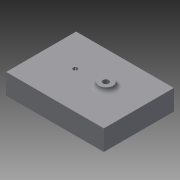
# Autodesk Inventor part: GehäuseFront
Saved by Autodesk Inventor 2014 (Build 180170000, 170)
## iProperties
Created: 2013-05-31
Part Number: GehäuseFront
Material: Generisch
Document SubType Name: Modeling
Designer: hanse
Density: 1 g/cm^3
Appearance: Vorgabe
Author: hanse
Autodesk Inventor part; units mm, degrees
ref_plane "YZ Plane" through (0, 0, 0) normal (1, 0, 0) x (0, 1, 0)
ref_plane "XZ Plane" through (0, 0, 0) normal (0, 1, 0) x (-1, 0, 0)
ref_plane "XY Plane" through (0, 0, 0) normal (0, 0, 1) x (1, 0, 0)
sketch "Skizze1" plane through (0, 0, 0) normal (0, 0, 1) x (1, 0, 0)
  line L0 (0, 0) -> (47.7997, 0)
  line L1 (47.7997, 0) -> (47.7997, 34.2455)
  line L2 (47.7997, 34.2455) -> (0, 34.2455)
  line L3 (0, 34.2455) -> (0, 0)
  circle A0 centre (15.5546, 18.2455) radius 1.05
  circle A1 centre (30.5546, 18.2455) radius 1.45
  line L4 (0, 18.2455) -> (47.7997, 18.2455)
  dimension "d0" = 2.1
  dimension "d1" = 2.9
  dimension "d2" = 15
  dimension "d16" = 16
  constraints: 10 end point, 4 point on line, 2 centre point, 2 parallel, 2 perpendicular, 1 horizontal
  measures "d0" diameter of A0
  measures "d1" diameter of A1
  measures "d2" distance of A1.centre A0.centre
  measures "d16" distance between parallel lines of L2 L4
extrude "Extrusion1" add sketch "Skizze1" along normal blind 2 contours L3 L4 A0 A1 L1 L0 | L3 L2 L1 L4 A1 A0
sketch "Skizze2" plane through (0, 0, 0) normal (0, 0, -1) x (-1, 0, 0)
  line L0 (0, 0) -> (-47.7997, 0) projected
  line L1 (0, 34.2455) -> (0, 0) projected
  line L2 (-47.7997, 34.2455) -> (0, 34.2455) projected
  line L3 (-47.7997, 0) -> (-47.7997, 34.2455) projected
  line L4 (-45.7997, 2) -> (-2, 2)
  line L5 (-2, 2) -> (-2, 32.2455)
  line L6 (-2, 32.2455) -> (-45.7997, 32.2455)
  line L7 (-45.7997, 32.2455) -> (-45.7997, 2)
  dimension "d5" = 2
  dimension "d6" = 2
  dimension "d7" = 2
  dimension "d8" = 2
  constraints: 8 end point, 2 parallel, 1 horizontal, 1 perpendicular
  measures "d5" distance between parallel lines of L2 L6
  measures "d6" distance between parallel lines of L5 L1
  measures "d7" distance between parallel lines of L3 L7
  measures "d8" distance between parallel lines of L0 L4
extrude "Extrusion2" add sketch "Skizze2" along normal blind 8
fillet "Rundung1" radius 2 8 edges at (23.8999, 0, 2) (47.7997, 0, -3) (47.7997, 17.1227, 2) (47.7997, 34.2455, -3) (23.8999, 34.2455, 2) (0, 17.1227, 2) (0, 34.2455, -3) (0, 0, -3)
sketch "Skizze3" plane through (0, 0, 0) normal (0, 0, -1) x (-1, 0, 0)
  circle A0 centre (-30.5546, 18.2455) radius 1.45 projected
  circle A1 centre (-30.5546, 18.2455) radius 2.95
  point P0 (0, 0)
  dimension "d12" = 1.5
  constraints: 1 centre point, 1 coincident
  measures "d12" radial gap between concentric circles of A0 A1
extrude "Extrusion3" add sketch "Skizze3" along normal blind 1
fillet "Rundung2" radius 2 1 edges at (33.5046, 18.2455, 0)
sketch "Skizze4" plane through (0, 0, 2) normal (0, 0, 1) x (1, 0, 0)
  circle A0 centre (30.5546, 18.2455) radius 1.45 projected
  circle A1 centre (30.5546, 18.2455) radius 3.45
  point P0 (0, 0)
  dimension "d17" = 2
  constraints: 1 centre point, 1 coincident
  measures "d17" radial gap between concentric circles of A0 A1
extrude "Extrusion4" add sketch "Skizze4" along normal blind 2
fillet "Rundung3" radius 2 1 edges at (27.1046, 18.2455, 2)
